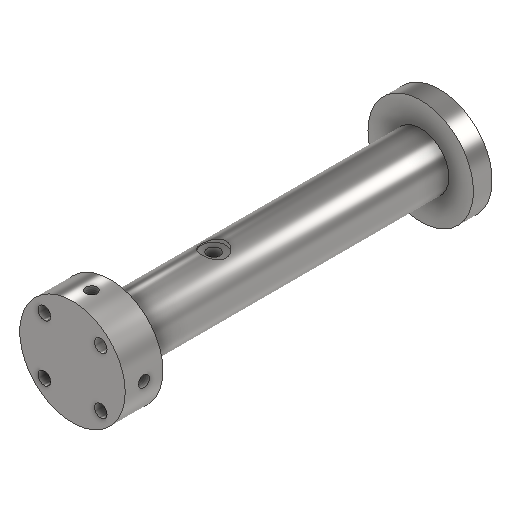
# Autodesk Inventor part: rotary_transfer_shaft_5_2
Saved by Autodesk Inventor 2026.2 (Build 302298000, 298)
## iProperties
Created: 2026-05-26
Part Number: rotary_transfer_shaft_5_2
Material: ステンレス鋼
Document SubType Name: Modeling
Designer: zetsu
Density: 8 g/cm^3
Appearance: 半つや出し
Author: zetsu
Autodesk Inventor part; units mm, degrees
sketch "スケッチ1" plane through (0, 0, 0) normal (0, 0, 1) x (1, 0, 0)
  circle A0 centre (0, 0) radius 7.5
  dimension "d0" = 15
  constraints: 1 centre point, 1 coincident
  measures "d0" diameter of A0
extrude "押し出し1" add sketch "スケッチ1" along normal blind 82.5
ref_plane "作業平面1" through (14, 0, 0) normal (1, 0, 0) x (0, 1, 0)
ref_plane "作業平面2" through (-14, 0, 0) normal (1, 0, 0) x (0, 1, 0)
ref_plane "作業平面3" through (0, 7.5, 0) normal (0, 1, 0) x (-1, 0, 0)
ref_plane "作業平面4" through (0, -7.5, 0) normal (0, 1, 0) x (-1, 0, 0)
sketch "スケッチ7" plane through (0, 7.5, 0) normal (0, 1, 0) x (-1, 0, 0)
  circle A0 centre (0, 55) radius 1.7
  line L0 (7.5, 82.5) -> (-7.5, 82.5) projected
  point P0 (0, 0)
  dimension "d35" = 3.4
  dimension "d87" = 27.5
  constraints: 1 centre point
  measures "d35" diameter of A0
  measures "d87" distance from line of L0 A0.centre
extrude "押し出し7" cut sketch "スケッチ7" against normal through all
sketch "スケッチ8" plane through (0, 7.5, 0) normal (0, 1, 0) x (-1, 0, 0)
  circle A0 centre (0, 55) radius 3.25
  line L0 (7.5, 82.5) -> (-7.5, 82.5) projected
  point P0 (0, 0)
  dimension "d39" = 6.5
  dimension "d85" = 27.5
  constraints: 1 centre point
  measures "d39" diameter of A0
  measures "d85" distance from line of L0 A0.centre
sketch "スケッチ9" plane through (0, -7.5, 0) normal (0, 1, 0) x (-1, 0, 0)
  circle A0 centre (0, 55) radius 3.25
  line L0 (7.5, 82.5) -> (-7.5, 82.5) projected
  point P0 (0, 0)
  dimension "d41" = 6.5
  dimension "d86" = 27.5
  constraints: 1 centre point
  measures "d41" diameter of A0
  measures "d86" distance from line of L0 A0.centre
extrude "押し出し8" cut sketch "スケッチ8" against normal blind 1
extrude "押し出し9" cut sketch "スケッチ9" along normal blind 1
sketch "スケッチ10" plane through (0, 0, 82.5) normal (0, 0, 1) x (1, 0, 0)
  circle A0 centre (0, 0) radius 14
  dimension "d47" = 28
  constraints: 1 centre point, 1 coincident
  measures "d47" diameter of A0
extrude "押し出し10" add sketch "スケッチ10" along normal blind 10
ref_plane "作業平面5" through (0, 14, 0) normal (0, 1, 0) x (-1, 0, 0)
ref_plane "作業平面6" through (0, -14, 0) normal (0, 1, 0) x (-1, 0, 0)
sketch "スケッチ11" plane through (0, 14, 0) normal (0, 1, 0) x (-1, 0, 0)
  circle A0 centre (0, 87.5) radius 1.5
  line L0 (14, 92.5) -> (-14, 92.5) projected
  point P0 (0, 0)
  dimension "d52" = 3
  dimension "d53" = 5
  constraints: 1 centre point
  measures "d52" diameter of A0
  measures "d53" distance from line of A0.centre L0
sketch "スケッチ12" plane through (0, -14, 0) normal (0, 1, 0) x (-1, 0, 0)
  circle A0 centre (0, 87.5) radius 1.5
  line L0 (14, 92.5) -> (-14, 92.5) projected
  point P0 (0, 0)
  dimension "d54" = 3
  dimension "d55" = 5
  constraints: 1 centre point
  measures "d54" diameter of A0
  measures "d55" distance from line of A0.centre L0
sketch "スケッチ13" plane through (-14, 0, 0) normal (1, 0, 0) x (0, 1, 0)
  circle A0 centre (0, 87.5) radius 1.5
  line L0 (14, 92.5) -> (-14, 92.5) projected
  point P0 (0, 0)
  dimension "d56" = 3
  dimension "d57" = 5
  constraints: 1 centre point
  measures "d56" diameter of A0
  measures "d57" distance from line of A0.centre L0
sketch "スケッチ14" plane through (14, 0, 0) normal (1, 0, 0) x (0, 1, 0)
  circle A0 centre (0, 87.5) radius 1.5
  line L0 (14, 92.5) -> (-14, 92.5) projected
  point P0 (0, 0)
  dimension "d58" = 3
  dimension "d59" = 5
  constraints: 1 centre point
  measures "d58" diameter of A0
  measures "d59" distance from line of A0.centre L0
extrude "押し出し11" cut sketch "スケッチ11" against normal blind 10
extrude "押し出し12" cut sketch "スケッチ12" along normal blind 10
extrude "押し出し13" cut sketch "スケッチ14" against normal blind 10
extrude "押し出し14" cut sketch "スケッチ13" along normal blind 10
thread "ねじ5" size "M3x0.5" class "6H" standard "ANSI Metric M Profile" full length
thread "ねじ6" size "M3x0.5" class "6H" standard "ANSI Metric M Profile" full length
thread "ねじ7" size "M3x0.5" class "6H" standard "ANSI Metric M Profile" full length
thread "ねじ8" size "M3x0.5" class "6H" standard "ANSI Metric M Profile" full length
sketch "スケッチ15" plane through (0, 0, 92.5) normal (0, 0, 1) x (1, 0, 0)
  circle A0 centre (7.5, 7.5) radius 1.7
  circle A1 centre (-7.5, 7.5) radius 1.7
  circle A2 centre (-7.5, -7.5) radius 1.7
  circle A3 centre (7.5, -7.5) radius 1.7
  point P0 (0, 0)
  dimension "d76" = 3.4
  dimension "d77" = 7.5
  dimension "d78" = 7.5
  dimension "d81" = 360
  constraints: 4 centre point, 9 other
  measures "d76" diameter of A0
  measures "d77" horizontal distance of A0.centre point (0, 0)
  measures "d78" horizontal distance of point (0, 0) A0.centre
extrude "押し出し15" cut sketch "スケッチ15" against normal through all
sketch "スケッチ16" plane through (0, 0, 0) normal (0, 0, -1) x (-1, 0, 0)
  circle A0 centre (0, 0) radius 14
  dimension "d88" = 28
  constraints: 1 centre point, 1 coincident
  measures "d88" diameter of A0
extrude "押し出し16" add sketch "スケッチ16" along normal blind 5
sketch "スケッチ17" plane through (0, 0, -5) normal (0, 0, -1) x (-1, 0, 0)
  arc A0 (-2.9394, 3) -> (2.9394, 3) centre (0, 0) ccw
  line L0 (-2.9394, 3) -> (2.9394, 3)
  dimension "d91" = 4.2
  dimension "d92" = 3
  constraints: 3 point on circle, 2 end point, 1 centre point, 1 coincident, 1 horizontal
  measures "d91" radius of A0
  measures "d92" distance from line of point (0, 0) L0
extrude "押し出し17" cut sketch "スケッチ17" against normal blind 80
